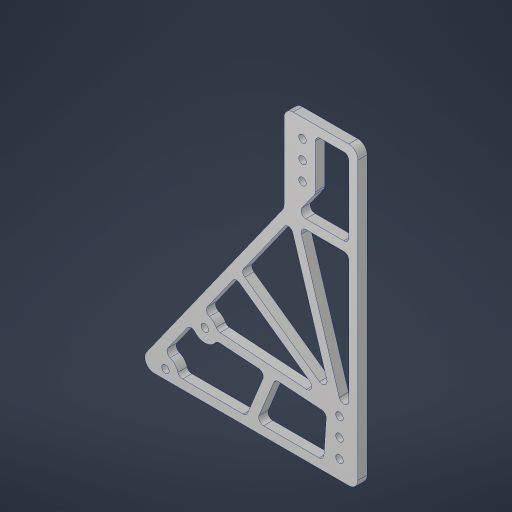
# Autodesk Inventor part: CL3-010
Saved by Autodesk Inventor 2023.4 (Build 274418000, 418)
## iProperties
RuleStatus: InUse
AfterDocNew0: SHOW
AfterDocOpen0: SHOW
Created: 2025-01-31
Part Number: CL3-010
Material: Aluminum 6061
Document SubType Name: Modeling
Designer: brand
Mass: 132.735 g
Surface Area: 177.419 cm^2
Volume: 49.1612 cm^3
Density: 2.7 g/cm^3
Appearance: Aluminum - Flat
Author: brand
Autodesk Inventor part; units mm, degrees
ref_plane "YZ Plane" through (0, 0, 0) normal (1, 0, 0) x (0, 1, 0)
ref_plane "XZ Plane" through (0, 0, 0) normal (0, 1, 0) x (-1, 0, 0)
ref_plane "XY Plane" through (0, 0, 0) normal (0, 0, 1) x (1, 0, 0)
sketch "Sketch1" plane through (0, 0, 0) normal (0, 0, 1) x (1, 0, 0)
  line L0 (-25.4, -101.6) -> (25.4, -101.6)
  line L1 (25.4, -101.6) -> (25.4, 101.6)
  line L2 (25.4, 101.6) -> (-25.4, 101.6)
  line L3 (-25.4, 101.6) -> (-25.4, -101.6)
  line L4 (-25.4, -101.6) -> (25.4, 101.6) construction
  line L5 (25.4, -101.6) -> (-25.4, 101.6) construction
  point P0 (0, 0)
  dimension "width" = 50.8
  dimension "length" = 203.2
  constraints: 12 end point, 2 midpoint, 2 parallel, 1 horizontal, 1 perpendicular
  measures "width" distance of L2.end L1.end
  measures "length" distance of L0.end L1.end
extrude "Extrusion1" add sketch "Sketch1" along normal mid plane 6.35
sketch "Sketch2" plane through (0, 0, 3.175) normal (0, 0, 1) x (1, 0, 0)
  line L0 (-25.4, -101.6) -> (-25.4, 101.6) construction
  line L1 (-25.4, 101.6) -> (25.4, 101.6) construction
  line L2 (25.4, 101.6) -> (25.4, -101.6) construction
  line L3 (25.4, -101.6) -> (-25.4, -101.6) construction
  point P0 (0, 0)
  point P1 (-12.7, 88.9)
  point P2 (-12.7, 76.2)
  point P3 (-12.7, 63.5)
  point P4 (12.7, -63.5)
  point P5 (12.7, -76.2)
  point P6 (12.7, -88.9)
  dimension "d4" = 25.4
  dimension "d5" = 12.7
  dimension "d6" = 12.7
  dimension "d7" = 12.7
  dimension "d8" = 12.7
  dimension "d9" = 12.7
  dimension "d10" = 12.7
  dimension "d11" = 25.4
  constraints: 4 vertical alignment
  measures "d4" distance from line of point (-12.7, 76.2) L1
  measures "d5" distance of point (-12.7, 76.2) point (-12.7, 88.9)
  measures "d6" distance of point (-12.7, 76.2) point (-12.7, 63.5)
  measures "d7" distance from line of L0 point (-12.7, 76.2)
  measures "d8" distance from line of L2 point (12.7, -76.2)
  measures "d9" distance of point (12.7, -63.5) point (12.7, -76.2)
  measures "d10" distance of point (12.7, -88.9) point (12.7, -76.2)
  measures "d11" distance from line of L3 point (12.7, -76.2)
hole "Hole1" at (-12.7, 88.9, 3.175) at (-12.7, 76.2, 3.175) at (-12.7, 63.5, 3.175) at (12.7, -63.5, 3.175) at (12.7, -76.2, 3.175) at (12.7, -88.9, 3.175) direction (0, 0, -1) diameter 5.1054 end through all clearance for "Flat Head Machine Screw (82)" size "#10" standard "Ansi Unified Screw Threads"
sketch "Sketch3" plane through (0, 0, 3.175) normal (0, 0, 1) x (1, 0, 0)
  circle A0 centre (12.7, -76.2) radius 2.5527 construction
  circle A1 centre (-12.7, 63.5) radius 2.5527 construction
  circle A2 centre (-12.7, 88.9) radius 2.5527 construction
  circle A3 centre (-12.7, 76.2) radius 2.5527 construction
  circle A4 centre (12.7, -63.5) radius 2.5527 construction
  circle A5 centre (12.7, -88.9) radius 2.5527 construction
  line L0 (-25.4, -101.6) -> (-25.4, 101.6) construction
  line L1 (-25.4, 101.6) -> (25.4, 101.6) construction
  line L2 (25.4, 101.6) -> (25.4, -101.6) construction
  line L3 (25.4, -101.6) -> (-25.4, -101.6) construction
  line L4 (-19.05, 95.25) -> (-19.05, -95.25) construction
  line L5 (-19.05, -95.25) -> (19.05, -95.25) construction
  line L6 (19.05, -95.25) -> (19.05, 95.25) construction
  line L7 (19.05, 95.25) -> (-19.05, 95.25) construction
  line L8 (-19.05, -95.25) -> (19.05, 95.25) construction
  line L9 (-19.05, 95.25) -> (19.05, -95.25) construction
  line L10 (-19.05, 0) -> (19.05, 0) construction
  line L11 (-19.05, -3.175) -> (19.05, -3.175) construction
  line L12 (-19.05, 3.175) -> (19.05, 3.175) construction
  circle A6 centre (-12.7, 63.5) radius 8.9027 construction
  circle A7 centre (-12.7, 76.2) radius 8.9027 construction
  circle A8 centre (-12.7, 88.9) radius 8.9027 construction
  circle A9 centre (12.7, -63.5) radius 8.9027 construction
  circle A10 centre (12.7, -76.2) radius 8.9027 construction
  circle A11 centre (12.7, -88.9) radius 8.9027 construction
  line L13 (3.7973, -63.5) -> (3.7973, -95.25) construction
  line L14 (12.7, -54.5973) -> (19.05, -54.5973) construction
  line L15 (-12.7, 54.5973) -> (-19.05, 54.5973) construction
  line L16 (-3.7973, 63.5) -> (-3.7973, 95.25) construction
  line L17 (15.8121, 95.25) -> (-19.05, -79.0606) construction
  line L18 (-15.8121, -95.25) -> (19.05, 79.0606) construction
  line L19 (-14.1573, 54.5973) -> (7.9555, -55.9669) construction
  line L20 (-7.9555, 55.9669) -> (14.1573, -54.5973) construction
  line L21 (-19.05, 54.5973) -> (-19.05, 3.175)
  line L22 (-19.05, 3.175) -> (-3.8729, 3.175)
  line L23 (-3.8729, 3.175) -> (-14.1573, 54.5973)
  line L24 (-14.1573, 54.5973) -> (-19.05, 54.5973)
  line L25 (3.8729, 3.175) -> (19.05, 3.175)
  line L26 (19.05, 3.175) -> (19.05, 79.0606)
  line L27 (19.05, 79.0606) -> (3.8729, 3.175)
  point P0 (0, 0)
  dimension "d19" = 6.35
  dimension "d20" = 3.175
  dimension "d21" = 3.175
  dimension "d22" = 6.35
  dimension "d23" = 6.35
  dimension "d24" = 6.35
  dimension "d25" = 6.35
  dimension "d26" = 6.35
  dimension "d27" = 6.35
  dimension "d28" = 3.175
  dimension "d29" = 3.175
  dimension "d30" = 3.175
  dimension "d31" = 3.175
  constraints: 48 end point, 23 point on line, 7 parallel, 6 centre point, 6 perpendicular, 6 point on circle, 4 tangent, 2 midpoint, 1 horizontal, 1 vertical, 3 other
  measures "d19" distance between parallel lines of L0 L4
  measures "d20" distance between parallel lines of L10 L11
  measures "d21" distance between parallel lines of L10 L12
  measures "d22" radial gap between concentric circles of A1 A6
  measures "d23" radial gap between concentric circles of A3 A7
  measures "d24" radial gap between concentric circles of A2 A8
  measures "d25" radial gap between concentric circles of A4 A9
  measures "d26" radial gap between concentric circles of A0 A10
  measures "d27" radial gap between concentric circles of A5 A11
  measures "d28" distance between parallel lines of L8 L17
  measures "d29" distance between parallel lines of L18 L8
  measures "d30" distance between parallel lines of L20 L9
  measures "d31" distance between parallel lines of L9 L19
sketch "Sketch4" plane through (0, 0, 3.175) normal (0, 0, 1) x (1, 0, 0)
  circle A0 centre (12.7, -76.2) radius 2.5527 construction
  circle A1 centre (-12.7, 63.5) radius 2.5527 construction
  circle A2 centre (-12.7, 88.9) radius 2.5527 construction
  circle A3 centre (-12.7, 76.2) radius 2.5527 construction
  circle A4 centre (12.7, -63.5) radius 2.5527 construction
  circle A5 centre (12.7, -88.9) radius 2.5527 construction
  line L0 (-25.4, -101.6) -> (-25.4, 101.6) construction
  line L1 (-25.4, 101.6) -> (25.4, 101.6) construction
  line L2 (25.4, 101.6) -> (25.4, -101.6) construction
  line L3 (25.4, -101.6) -> (-25.4, -101.6) construction
  line L4 (25.4, -101.6) -> (-127, -101.6) construction
  line L5 (-127, -101.6) -> (-127, -50.8) construction
  line L6 (-127, -50.8) -> (25.4, -50.8) construction
  line L7 (25.4, -50.8) -> (25.4, -101.6) construction
  line L8 (-127, -101.6) -> (-25.4, -101.6)
  line L9 (-25.4, -101.6) -> (-25.4, 101.6)
  line L10 (-25.4, 41.275) -> (-127, -101.6)
  circle A6 centre (-100.7141, -86.5499) radius 4.7625 construction
  circle A7 centre (-85.9941, -65.8501) radius 4.7625 construction
  line L11 (-100.7141, -86.5499) -> (-85.9941, -65.8501) construction
  point P0 (0, 0)
  point P1 (-127, -76.2)
  point P2 (-93.3541, -76.2)
  dimension "d32" = 50.8
  dimension "d33" = 152.4
  dimension "d36" = 9.525
  dimension "d37" = 9.525
  dimension "d38" = 12.7
  dimension "d39" = 25.4
  dimension "d47" = 60.325
  constraints: 16 end point, 3 parallel, 2 centre point, 2 horizontal, 2 midpoint, 2 perpendicular, 1 horizontal alignment, 1 point on line
  measures "d32" distance of L4.end L5.end
  measures "d33" distance between parallel lines of L2 L5
  measures "d36" diameter of A6
  measures "d37" diameter of A7
  measures "d38" distance between parallel lines of L10 L11
  measures "d39" distance of L11.start L11.end
  measures "d47" distance from line of L1 L10.start
extrude "Extrusion2" add sketch "Sketch4" against normal up to surface (6.35 mm away)
sketch "Sketch5" plane through (0, 0, 3.175) normal (0, 0, 1) x (1, 0, 0)
  line L0 (-127, -101.6) -> (25.4, -101.6) construction
  line L1 (25.4, -101.6) -> (-228.6, -101.6) construction
  line L2 (-228.6, -101.6) -> (-228.6, -50.8) construction
  line L3 (-228.6, -50.8) -> (25.4, -50.8) construction
  line L4 (25.4, -50.8) -> (25.4, -101.6) construction
  line L5 (23.8125, -52.3875) -> (-227.0125, -52.3875) construction
  line L6 (-227.0125, -52.3875) -> (-227.0125, -100.0125) construction
  line L7 (-227.0125, -100.0125) -> (23.8125, -100.0125) construction
  line L8 (23.8125, -100.0125) -> (23.8125, -52.3875) construction
  circle A0 centre (-79.8345, -57.1881) radius 4.8006 construction
  circle A1 centre (-106.8737, -95.2119) radius 4.8006 construction
  line L9 (-106.8737, -95.2119) -> (-79.8345, -57.1881) construction
  circle A2 centre (12.7, -76.2) radius 2.5527 construction
  circle A3 centre (-12.7, 63.5) radius 2.5527 construction
  circle A4 centre (-12.7, 88.9) radius 2.5527 construction
  circle A5 centre (-12.7, 76.2) radius 2.5527 construction
  circle A6 centre (12.7, -63.5) radius 2.5527 construction
  circle A7 centre (12.7, -88.9) radius 2.5527 construction
  line L10 (-127, -101.6) -> (25.4, -101.6) construction
  line L11 (25.4, -101.6) -> (25.4, 101.6) construction
  line L12 (25.4, 101.6) -> (-25.4, 101.6) construction
  line L13 (-25.4, 101.6) -> (-25.4, 41.275) construction
  line L14 (-25.4, 41.275) -> (-127, -101.6) construction
  point P0 (0, 0)
  point P1 (-93.3541, -76.2)
  dimension "d48" = 254
  dimension "d49" = 50.8
  dimension "d50" = 1.5875
  dimension "d51" = 9.6012
  dimension "d52" = 12.7
  constraints: 18 end point, 5 parallel, 2 centre point, 2 coincident, 2 perpendicular, 2 tangent, 1 equal radius, 1 horizontal, 1 midpoint, 3 other
  measures "d48" distance of L2.end L3.end
  measures "d49" distance of L1.end L2.end
  measures "d50" distance between parallel lines of L3 L5
  measures "d51" diameter of A0
  measures "d52" distance from line of L14 point (-93.354, -76.2)
hole "Hole2" at (-79.8345, -57.1881, 3.175) at (-106.8737, -95.2119, 3.175) direction (0, 0, -1) diameter 5.1054 end through all clearance for "Flat Head Machine Screw (82)" size "#10" standard "Ansi Unified Screw Threads"
sketch "Sketch6" plane through (0, 0, 3.175) normal (0, 0, 1) x (1, 0, 0)
  circle A0 centre (-79.8345, -57.1881) radius 2.5527 construction
  circle A1 centre (-106.8737, -95.2119) radius 2.5527 construction
  line L0 (-127, -101.6) -> (-25.4, 41.275) construction
  line L1 (-25.4, 41.275) -> (-25.4, 101.6) construction
  line L2 (-25.4, 101.6) -> (25.4, 101.6) construction
  line L3 (25.4, 101.6) -> (25.4, -101.6) construction
  line L4 (25.4, -101.6) -> (-127, -101.6) construction
  circle A2 centre (12.7, -76.2) radius 2.5527 construction
  circle A3 centre (-12.7, 63.5) radius 2.5527 construction
  circle A4 centre (-12.7, 88.9) radius 2.5527 construction
  circle A5 centre (-12.7, 76.2) radius 2.5527 construction
  circle A6 centre (12.7, -63.5) radius 2.5527 construction
  circle A7 centre (12.7, -88.9) radius 2.5527 construction
  line L5 (19.05, 95.25) -> (-19.05, 95.25) construction
  line L6 (-19.05, 95.25) -> (-19.05, 39.2474) construction
  line L7 (-5.8315, 57.8359) -> (-114.6926, -95.25) construction
  line L8 (-114.6926, -95.25) -> (19.05, -95.25) construction
  line L9 (19.05, -95.25) -> (19.05, 95.25) construction
  circle A8 centre (-12.7, 88.9) radius 8.9027 construction
  circle A9 centre (-12.7, 76.2) radius 8.9027 construction
  circle A10 centre (-12.7, 63.5) radius 8.9027 construction
  circle A11 centre (12.7, -63.5) radius 8.9027 construction
  circle A12 centre (12.7, -76.2) radius 8.9027 construction
  circle A13 centre (12.7, -88.9) radius 8.9027 construction
  circle A14 centre (-79.8345, -57.1881) radius 8.9027 construction
  circle A15 centre (-106.8737, -95.2119) radius 8.9027 construction
  circle A16 centre (-79.8345, -57.1881) radius 2.5527 construction
  line L10 (-79.8345, -57.1881) -> (12.7, -63.5) construction
  line L11 (-3.7973, 63.5) -> (-3.7973, 95.25) construction
  line L12 (3.7973, -63.5) -> (3.7973, -95.25) construction
  line L13 (-87.9165, -53.4544) -> (21.2141, -60.8984) construction
  line L14 (-71.7526, -60.9218) -> (4.1859, -66.1016) construction
  line L15 (-47.8213, -95.25) -> (-33.5673, -60.3441) construction
  circle A17 centre (12.7, -63.5) radius 2.5527 construction
  line L16 (-19.05, 39.2474) -> (12.7, -63.5) construction
  line L17 (-19.05, 50.0015) -> (15.0901, -60.4807) construction
  line L18 (-21.3665, 35.9898) -> (8.3008, -60.0175) construction
  line L19 (12.7, -63.5) -> (-56.913, -13.9974) construction
  line L20 (-58.753, -16.5849) -> (1.69, -59.5666) construction
  line L21 (-55.073, -11.4099) -> (7.7618, -56.0924) construction
  line L22 (-31.495, -63.6678) -> (-44.3918, -95.25) construction
  line L23 (-38.1682, -63.2126) -> (-51.2508, -95.25) construction
  line L24 (-19.05, 39.2474) -> (19.05, 39.2474) construction
  line L25 (-14.7458, 36.0724) -> (19.05, 36.0724) construction
  line L26 (-16.7922, 42.4224) -> (19.05, 42.4224) construction
  line L27 (-97.9711, -95.25) -> (-51.2508, -95.25)
  line L28 (-51.2508, -95.25) -> (-38.1682, -63.2126)
  line L29 (-38.1682, -63.2126) -> (-71.7526, -60.9218)
  line L30 (-108.4325, -86.4467) -> (-88.6256, -58.5933)
  arc A18 (-88.6256, -58.5933) -> (-71.7526, -60.9218) centre (-79.8345, -57.1881) ccw
  arc A19 (-97.9711, -95.25) -> (-108.4325, -86.4467) centre (-106.8737, -95.2119) ccw
  line L31 (1.8072, -95.25) -> (-44.3918, -95.25)
  line L32 (-44.3918, -95.25) -> (-31.495, -63.6678)
  line L33 (-31.495, -63.6678) -> (3.7973, -66.0751)
  line L34 (3.7973, -66.0751) -> (1.8072, -95.25)
  line L35 (-58.753, -16.5849) -> (-81.3934, -48.4229)
  line L36 (-58.753, -16.5849) -> (1.69, -59.5666)
  line L37 (1.69, -59.5666) -> (-71.3204, -54.5865)
  arc A20 (-71.3204, -54.5865) -> (-81.3934, -48.4229) centre (-79.8345, -57.1881) ccw
  line L38 (-55.073, -11.4099) -> (-21.3665, 35.9898)
  line L39 (-21.3665, 35.9898) -> (6.8981, -55.4783)
  line L40 (6.8981, -55.4783) -> (-55.073, -11.4099)
  line L41 (-14.7458, 36.0724) -> (19.05, 36.0724)
  line L42 (19.05, 36.0724) -> (19.05, -73.2954)
  line L43 (19.05, -73.2954) -> (-14.7458, 36.0724)
  line L44 (-16.7922, 42.4224) -> (19.05, 42.4224)
  line L45 (19.05, 42.4224) -> (19.05, 95.25)
  line L46 (19.05, 95.25) -> (-3.7973, 95.25)
  line L47 (-3.7973, 95.25) -> (-3.7973, 60.6965)
  line L48 (-3.7973, 60.6965) -> (-16.7922, 42.4224)
  point P0 (0, 0)
  dimension "off" = 6.35
  dimension "d54" = 6.35
  dimension "d55" = 6.35
  dimension "d56" = 6.35
  dimension "d57" = 6.35
  dimension "d58" = 6.35
  dimension "d59" = 6.35
  dimension "d60" = 6.35
  dimension "d61" = 6.35
  dimension "d62" = 3.175
  dimension "d63" = 3.175
  dimension "d64" = 3.175
  dimension "d65" = 3.175
  dimension "d66" = 6.35
  dimension "d67" = 6.35
  dimension "d68" = 3.175
  dimension "d69" = 6.35
  dimension "d70" = 3.175
  dimension "d71" = 6.35
  dimension "d72" = 3.175
  dimension "d73" = 6.35
  constraints: 88 end point, 41 point on line, 16 point on circle, 11 centre point, 8 parallel, 7 perpendicular, 6 horizontal, 4 tangent, 2 coincident, 2 midpoint, 1 horizontal alignment, 20 other
  measures "off" distance between parallel lines of L2 L5
  measures "d54" radial gap between concentric circles of A4 A8
  measures "d55" radial gap between concentric circles of A5 A9
  measures "d56" radial gap between concentric circles of A3 A10
  measures "d57" radial gap between concentric circles of A6 A11
  measures "d58" radial gap between concentric circles of A2 A12
  measures "d59" radial gap between concentric circles of A7 A13
  measures "d60" radial gap between concentric circles of A0 A14
  measures "d61" radial gap between concentric circles of A1 A15
  measures "d62" distance between parallel lines of L10 L13
  measures "d63" distance between parallel lines of L10 L14
  measures "d64" distance between parallel lines of L16 L17
  measures "d65" distance between parallel lines of L16 L18
  measures "d67" distance between parallel lines of L3 L9
  measures "d68" distance between parallel lines of L19 L21
  measures "d69" distance between parallel lines of L20 L21
  measures "d70" distance between parallel lines of L15 L22
  measures "d71" distance between parallel lines of L23 L22
  measures "d72" distance between parallel lines of L26 L24
  measures "d73" distance between parallel lines of L25 L26
extrude "Extrusion3" cut sketch "Sketch6" against normal through all
fillet "Fillet1" radius 6.35 5 edges at (-127, -101.6, 0) (25.4, -101.6, 0) (-25.4, 41.275, 0) (-25.4, 101.6, 0) (25.4, 101.6, 0)
fillet "Fillet2" radius 3.302 25 edges at (1.69, -59.5666, 0) (-58.753, -16.5849, 0) (-81.3934, -48.4229, 0) (-71.3204, -54.5865, 0) (-16.7922, 42.4224, 0) (19.05, 42.4224, 0) (19.05, 95.25, 0) (-3.7973, 95.25, 0) (-3.7973, 60.6965, 0) (-88.6256, -58.5933, 0) (-108.4325, -86.4467, 0) (-97.9711, -95.25, 0) (-51.2508, -95.25, 0) (-38.1682, -63.2126, 0) (-71.7526, -60.9218, 0) (6.8981, -55.4783, 0) (-21.3665, 35.9898, 0) (-55.073, -11.4099, 0) (19.05, -73.2954, 0) (19.05, 36.0724, 0) (-14.7458, 36.0724, 0) (1.8072, -95.25, 0) (3.7973, -66.0751, 0) (-31.495, -63.6678, 0) (-44.3918, -95.25, 0)
equation "\"d6\" = d5"
equation "\"d8\" = d7"
equation "\"d9\" = d5"
equation "\"d10\" = d9"
equation "\"d11\" = d4"
equation "\"d20\" = 0.5 * d19"
equation "\"d21\" = d20"
equation "\"d22\" = d19"
equation "\"d23\" = d19"
equation "\"d24\" = d19"
equation "\"d25\" = d19"
equation "\"d26\" = d19"
equation "\"d27\" = d19"
equation "\"d28\" = d21"
equation "\"d29\" = d28"
equation "\"d30\" = d20"
equation "\"d31\" = d30"
equation "\"d37\" = d36"
equation "\"d54\" = off"
equation "\"d55\" = off"
equation "\"d56\" = off"
equation "\"d57\" = off"
equation "\"d58\" = off"
equation "\"d59\" = off"
equation "\"d60\" = off"
equation "\"d61\" = off"
equation "\"d62\" = 0.5 * off"
equation "\"d63\" = 0.5 * off"
equation "\"d64\" = 0.5 * off"
equation "\"d65\" = 0.5 * off"
equation "\"d66\" = off"
equation "\"d67\" = off"
equation "\"d68\" = 0.5 * off"
equation "\"d69\" = off"
equation "\"d70\" = 0.5 * off"
equation "\"d71\" = off"
equation "\"d72\" = 0.5 * off"
equation "\"d73\" = off"
body "Solid1"
